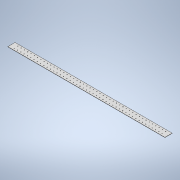
# Autodesk Inventor part: Assembly_plate_beamV3
Saved by Autodesk Inventor 2022 (Build 260153000, 153)
## iProperties
Created: 2022-04-25
Part Number: Assembly_plate_beamV3
Material: Generic
Document SubType Name: Sheet Metal
Designer: Patrick
Density: 1 g/cm^3
Sheet Metal Rule: Default_mm
Appearance: Default
Author: Patrick
Autodesk Inventor part; units mm, degrees
ref_plane "YZ Plane" through (0, 0, 0) normal (1, 0, 0) x (0, 1, 0)
ref_plane "XZ Plane" through (0, 0, 0) normal (0, 1, 0) x (-1, 0, 0)
ref_plane "XY Plane" through (0, 0, 0) normal (0, 0, 1) x (1, 0, 0)
sketch "Sketch1" plane through (0, 0, 0) normal (0, 1, 0) x (-1, 0, 0)
  line L0 (0, 0) -> (956, 0)
  line L1 (956, 0) -> (956, -44)
  line L2 (956, -44) -> (0, -44)
  line L3 (0, -44) -> (0, 0)
  circle A0 centre (928, -11) radius 1.675
  circle A1 centre (908, -11) radius 1.675
  circle A2 centre (888, -11) radius 1.675
  circle A3 centre (868, -11) radius 1.675
  circle A4 centre (848, -11) radius 1.675
  circle A5 centre (828, -11) radius 1.675
  circle A6 centre (808, -11) radius 1.675
  circle A7 centre (788, -11) radius 1.675
  circle A8 centre (768, -11) radius 1.675
  circle A9 centre (748, -11) radius 1.675
  circle A10 centre (728, -11) radius 1.675
  circle A11 centre (708, -11) radius 1.675
  circle A12 centre (688, -11) radius 1.675
  circle A13 centre (668, -11) radius 1.675
  circle A14 centre (648, -11) radius 1.675
  circle A15 centre (628, -11) radius 1.675
  circle A16 centre (608, -11) radius 1.675
  circle A17 centre (588, -11) radius 1.675
  circle A18 centre (568, -11) radius 1.675
  circle A19 centre (548, -11) radius 1.675
  circle A20 centre (528, -11) radius 1.675
  circle A21 centre (508, -11) radius 1.675
  circle A22 centre (488, -11) radius 1.675
  circle A23 centre (468, -11) radius 1.675
  circle A24 centre (448, -11) radius 1.675
  circle A25 centre (428, -11) radius 1.675
  circle A26 centre (408, -11) radius 1.675
  circle A27 centre (388, -11) radius 1.675
  circle A28 centre (368, -11) radius 1.675
  circle A29 centre (348, -11) radius 1.675
  circle A30 centre (328, -11) radius 1.675
  circle A31 centre (308, -11) radius 1.675
  circle A32 centre (288, -11) radius 1.675
  circle A33 centre (268, -11) radius 1.675
  circle A34 centre (248, -11) radius 1.675
  circle A35 centre (228, -11) radius 1.675
  circle A36 centre (208, -11) radius 1.675
  circle A37 centre (188, -11) radius 1.675
  circle A38 centre (168, -11) radius 1.675
  circle A39 centre (148, -11) radius 1.675
  circle A40 centre (128, -11) radius 1.675
  circle A41 centre (108, -11) radius 1.675
  circle A42 centre (88, -11) radius 1.675
  circle A43 centre (68, -11) radius 1.675
  circle A44 centre (48, -11) radius 1.675
  circle A45 centre (28, -11) radius 1.675
  circle A46 centre (928, -33) radius 1.675
  circle A47 centre (908, -33) radius 1.675
  circle A48 centre (888, -33) radius 1.675
  circle A49 centre (868, -33) radius 1.675
  circle A50 centre (848, -33) radius 1.675
  circle A51 centre (828, -33) radius 1.675
  circle A52 centre (808, -33) radius 1.675
  circle A53 centre (788, -33) radius 1.675
  circle A54 centre (768, -33) radius 1.675
  circle A55 centre (748, -33) radius 1.675
  circle A56 centre (728, -33) radius 1.675
  circle A57 centre (708, -33) radius 1.675
  circle A58 centre (688, -33) radius 1.675
  circle A59 centre (668, -33) radius 1.675
  circle A60 centre (648, -33) radius 1.675
  circle A61 centre (628, -33) radius 1.675
  circle A62 centre (608, -33) radius 1.675
  circle A63 centre (588, -33) radius 1.675
  circle A64 centre (568, -33) radius 1.675
  circle A65 centre (548, -33) radius 1.675
  circle A66 centre (528, -33) radius 1.675
  circle A67 centre (508, -33) radius 1.675
  circle A68 centre (488, -33) radius 1.675
  circle A69 centre (468, -33) radius 1.675
  circle A70 centre (448, -33) radius 1.675
  circle A71 centre (428, -33) radius 1.675
  circle A72 centre (408, -33) radius 1.675
  circle A73 centre (388, -33) radius 1.675
  circle A74 centre (368, -33) radius 1.675
  circle A75 centre (348, -33) radius 1.675
  circle A76 centre (328, -33) radius 1.675
  circle A77 centre (308, -33) radius 1.675
  circle A78 centre (288, -33) radius 1.675
  circle A79 centre (268, -33) radius 1.675
  circle A80 centre (248, -33) radius 1.675
  circle A81 centre (228, -33) radius 1.675
  circle A82 centre (208, -33) radius 1.675
  circle A83 centre (188, -33) radius 1.675
  circle A84 centre (168, -33) radius 1.675
  circle A85 centre (148, -33) radius 1.675
  circle A86 centre (128, -33) radius 1.675
  circle A87 centre (108, -33) radius 1.675
  circle A88 centre (88, -33) radius 1.675
  circle A89 centre (68, -33) radius 1.675
  circle A90 centre (48, -33) radius 1.675
  circle A91 centre (28, -33) radius 1.675
  dimension "d0" = 44
  dimension "d1" = 956
  dimension "d2" = 11
  dimension "d3" = 28
  dimension "d4" = 3.35
  dimension "d7" = 20
  dimension "d10" = 22
  measures "d0" distance of L2.end L0.start
  measures "d1" distance of L1.end L2.end
  measures "d2" distance from line of L0 A0.centre
  measures "d3" distance from line of L1 A0.centre
  measures "d4" diameter of A0
  measures "d7" distance of A0.centre A1.centre
  measures "d10" distance of A0.centre A46.centre
extrude "Plate2" add sketch "Sketch1" along normal blind 1.5
equation "\"d14\" = Thickness"
equation "\"BendRadius\" = Thickness"
equation "\"BendReliefWidth\" = Thickness"
equation "\"BendReliefDepth\" = 0.5 * Thickness"
equation "\"CornerReliefSize\" = 4 * Thickness"
equation "\"MinimumRemnant\" = 2 * Thickness"
equation "\"TransitionRadius\" = BendRadius"
equation "\"JacobiRadiusSize\" = BendRadius"
equation "\"GapSize\" = Thickness"
equation "\"Thickness\" = 1.5"
body "Solid2"
